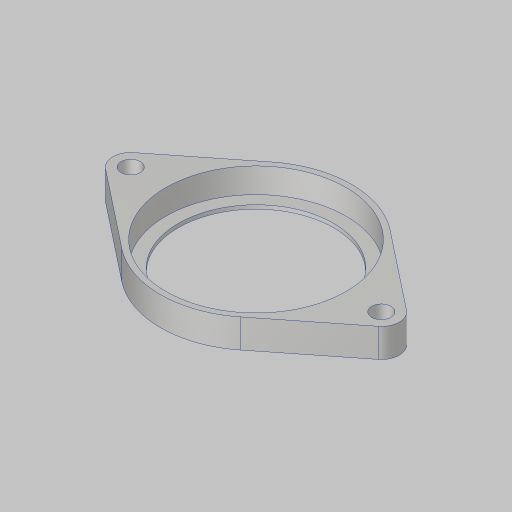
# Autodesk Inventor part: EL2-CGB-008
Saved by Autodesk Inventor 2023.5 (Build 275446000, 446)
## iProperties
Created: 2025-01-24
Part Number: EL2-CGB-008
Material: Aluminum 6061
Document SubType Name: Modeling
Designer: slick
Density: 2.7 g/cm^3
Appearance: Aluminum - Flat
Author: slick
Autodesk Inventor part; units mm, degrees
ref_plane "YZ Plane" through (0, 0, 0) normal (1, 0, 0) x (0, 1, 0)
ref_plane "XZ Plane" through (0, 0, 0) normal (0, 1, 0) x (-1, 0, 0)
ref_plane "XY Plane" through (0, 0, 0) normal (0, 0, 1) x (1, 0, 0)
sketch "Sketch1" plane through (0, 0, 0) normal (0, 1, 0) x (-1, 0, 0)
  circle A0 centre (0, 0) radius 23.8125 construction
  line L0 (33.3248, 0) -> (-33.3248, 0) construction
  circle A1 centre (33.3248, 0) radius 4.7625 construction
  circle A2 centre (-33.3248, 0) radius 4.7625 construction
  circle A3 centre (0, 0) radius 20.6375
  circle A4 centre (0, 0) radius 25.4 construction
  line L1 (36.2741, 3.7394) -> (15.7298, 19.9433)
  line L2 (36.2741, -3.7394) -> (15.7298, -19.9433)
  line L3 (-15.7298, -19.9433) -> (-36.2741, -3.7394)
  line L4 (-36.2741, 3.7394) -> (-15.7298, 19.9433)
  arc A5 (15.7298, 19.9433) -> (-15.7298, 19.9433) centre (0, 0) ccw
  arc A6 (-15.7298, -19.9433) -> (15.7298, -19.9433) centre (0, 0) ccw
  arc A7 (36.2741, -3.7394) -> (36.2741, 3.7394) centre (33.3248, 0) ccw
  arc A8 (-36.2741, 3.7394) -> (-36.2741, -3.7394) centre (-33.3248, 0) ccw
  point P0 (-36.2741, -3.7394)
  dimension "d0" = 47.625
  dimension "d1" = 33.3248
  dimension "d2" = 9.525
  dimension "d3" = 3.175
  dimension "d4" = 1.5875
  constraints: 17 point on circle, 10 end point, 9 centre point, 8 tangent, 7 coincident, 2 equal radius, 2 midpoint, 1 horizontal
  measures "d0" diameter of A0
  measures "d1" distance of L0.start point (0, 0)
  measures "d2" diameter of A1
  measures "d3" radial gap between concentric circles of A0 A3
  measures "d4" radial gap between concentric circles of A0 A4
extrude "Extrusion1" add sketch "Sketch1" along normal blind 7.62
sketch "Sketch2" plane through (0, 7.62, 0) normal (0, 1, 0) x (1, 0, 0)
  circle A0 centre (0, 0) radius 23.9395
  dimension "d7" = 47.879
  constraints: 1 centre point, 1 coincident
  measures "d7" diameter of A0
extrude "Extrusion2" cut sketch "Sketch2" against normal blind 6.604
hole "Hole1" at (-33.3248, 0, 0) at (33.3248, 0, 0) direction (0, 1, 0) diameter 5.1054 end through all clearance for "Flat Head Machine Screw (82)" size "#10" standard "Ansi Unified Screw Threads"
body "Solid1"
